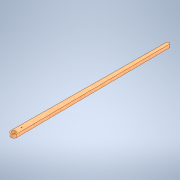
# Autodesk Inventor part: arm
Saved by Autodesk Inventor 2021 (Build 250183000, 183)
## iProperties
Created: 2021-07-07
Part Number: arm
Material: Wood (Cherry)
Document SubType Name: Modeling
Designer: KAVYA
Density: 0.63 g/cm^3
Appearance: Cherry - Natural Low Gloss
Author: KAVYA
Autodesk Inventor part; units mm, degrees
ref_plane "YZ Plane" through (0, 0, 0) normal (1, 0, 0) x (0, 1, 0)
ref_plane "XZ Plane" through (0, 0, 0) normal (0, 1, 0) x (-1, 0, 0)
ref_plane "XY Plane" through (0, 0, 0) normal (0, 0, 1) x (1, 0, 0)
sketch "Sketch1" plane through (0, 0, 0) normal (0, 1, 0) x (-1, 0, 0)
  arc A0 (2.9205, -0.0553) -> (-2.9205, -0.0553) centre (0, 0) ccw
  arc A1 (-1.5, -150) -> (1.5, -150) centre (0, -150) ccw
  line L0 (2.921, 0) -> (1.5, -150)
  line L1 (-2.921, 0) -> (-1.5, -150)
  dimension "d1" = 5.842
  dimension "d3" = 3
  constraints: 6 point on circle, 4 end point, 2 centre point, 2 point on line, 1 coincident
  measures "d1" diameter of A0
  measures "d3" diameter of A1
extrude "Extrusion1" add sketch "Sketch1" along normal blind 3
sketch "Sketch2" plane through (0, 3, 0) normal (0, 1, 0) x (1, 0, 0)
  circle A0 centre (0, 0) radius 1.905
  dimension "d6" = 3.81
  constraints: 1 centre point, 1 coincident
  measures "d6" diameter of A0
extrude "Extrusion2" cut sketch "Sketch2" against normal blind 3
sketch "Sketch3" plane through (0, 3, 0) normal (0, 1, 0) x (1, 0, 0)
  circle A0 centre (0, 7.62) radius 0.381
  point P0 (0, 0)
  dimension "d10" = 0.762
  constraints: 1 centre point
  measures "d10" diameter of A0
extrude "Extrusion3" cut sketch "Sketch3" against normal blind 3
body "Solid1"
